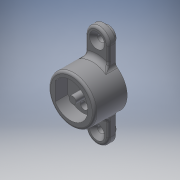
# Autodesk Inventor part: cycloid_input_cam_motor_adapter
Saved by Autodesk Inventor 2019.4 (Build 234330000, 330)
## iProperties
Created: 2019-09-11
Part Number: cycloid_input_cam_motor_adapter
Material: Generic
Document SubType Name: Modeling
Designer: cdi
Density: 1 g/cm^3
Appearance: Default
Author: cdi
Autodesk Inventor part; units mm, degrees
ref_plane "YZ Plane" through (0, 0, 0) normal (1, 0, 0) x (0, 1, 0)
ref_plane "XZ Plane" through (0, 0, 0) normal (0, 1, 0) x (-1, 0, 0)
ref_plane "XY Plane" through (0, 0, 0) normal (0, 0, 1) x (1, 0, 0)
sketch "Sketch1" plane through (0, 0, 0) normal (0, 0, 1) x (1, 0, 0)
  circle A0 centre (0, 0) radius 10
  dimension "d0" = 20
  constraints: 1 centre point, 1 coincident
  measures "d0" diameter of A0
extrude "Extrusion1" add sketch "Sketch1" along normal blind 8.5
sketch "Sketch2" plane through (0, 0, 8.5) normal (0, 0, 1) x (1, 0, 0)
  circle A0 centre (0, 0) radius 1.5
  dimension "d3" = 3
  constraints: 1 centre point, 1 coincident
  measures "d3" diameter of A0
extrude "Extrusion2" add sketch "Sketch2" along normal blind 5
chamfer "Chamfer1" distance 0.4 angle 45 1 edges at (-1.5, 0, 8.5)
sketch "Sketch3" plane through (0, 0, 8.5) normal (0, 0, 1) x (1, 0, 0)
  circle A0 centre (-0.5, 0) radius 7.575
  circle A1 centre (0, 0) radius 10 projected
  line L0 (0, 0) -> (-7.1422, 0)
  dimension "d9" = 15.15
  dimension "d25" = 0.5
  constraints: 2 end point, 1 centre point, 1 horizontal, 1 point on line
  measures "d9" diameter of A0
  measures "d25" distance of point (0, 0) A0.centre
extrude "Extrusion3" add sketch "Sketch3" along normal blind 5.5
sketch "Sketch4" plane through (0, 0, 0) normal (0, 0, -1) x (-1, 0, 0)
  circle A0 centre (0, 4.5) radius 1.5
  point P0 (0, 0)
  dimension "d13" = 4.5
  dimension "d14" = 3
  constraints: 1 centre point
  measures "d13" distance of point (0, 0) A0.centre
  measures "d14" diameter of A0
hole "Hole1" at (0, 4.5, 0) direction (0, 0, 1) diameter 3.25 end through all countersink diameter 6.5 countersink angle 90
pattern_circular "Circular Pattern1" count 2 over 360 about axis through (0, 0, 0) along (0, 0, 1) of "Hole1"
sketch "Sketch5" plane through (0, 0, 0) normal (0, 0, -1) x (-1, 0, 0)
  line L0 (-5, 17) -> (5, 17)
  line L1 (5, 17) -> (5, -17)
  line L2 (5, -17) -> (-5, -17)
  line L3 (-5, -17) -> (-5, 17)
  line L4 (-5, 17) -> (5, -17) construction
  line L5 (5, 17) -> (-5, -17) construction
  circle A0 centre (0, 0) radius 10 projected
  arc A1 (5, 8.6603) -> (-5, 8.6603) centre (0, 0) ccw
  arc A2 (-5, -8.6603) -> (5, -8.6603) centre (0, 0) ccw
  dimension "d26" = 10
  dimension "d27" = 34
  constraints: 12 end point, 8 point on circle, 4 point on line, 2 centre point, 2 concentric, 2 midpoint, 2 parallel, 1 horizontal, 1 perpendicular
  measures "d26" distance of L1.end L2.end
  measures "d27" distance of L0.end L1.end
extrude "Extrusion4" add sketch "Sketch5" against normal blind 3 contours L0 L1 A0 L3 | A0 L1 L2 L3
sketch "Sketch6" plane through (0, 0, 0) normal (0, 0, -1) x (-1, 0, 0)
  line L0 (-5, 17) -> (5, 17) projected
  circle A0 centre (0, 17) radius 5
  line L1 (5, -17) -> (-5, -17) projected
  circle A1 centre (0, -17) radius 5
  point P0 (0, 0)
  constraints: 2 horizontal alignment, 2 midpoint, 4 other
extrude "Extrusion5" add sketch "Sketch6" against normal blind 3
sketch "Sketch7" plane through (0, 0, 0) normal (0, 0, -1) x (-1, 0, 0)
  arc A0 (5, 17) -> (-5, 17) centre (0, 17) ccw projected
  circle A1 centre (0, 17) radius 3.25
  arc A2 (-5, -17) -> (5, -17) centre (0, -17) ccw projected
  circle A3 centre (0, -17) radius 3.25
  point P0 (0, 0)
  dimension "d32" = 6.5
  dimension "d33" = 6.5
  constraints: 2 centre point, 2 coincident
  measures "d32" diameter of A1
  measures "d33" diameter of A3
extrude "Extrusion6" add sketch "Sketch7" along normal blind 2
sketch "Sketch8" plane through (0, 0, 3) normal (0, 0, 1) x (1, 0, 0)
  arc A0 (5, 17) -> (-5, 17) centre (0, 17) ccw projected
  arc A1 (-5, -17) -> (5, -17) centre (0, -17) ccw projected
  point P0 (0, 0)
hole "Hole2" at (0, 17, 3) at (0, -17, 3) direction (0, 0, -1) diameter 3.1 end through all countersink diameter 6.5 countersink angle 90
fillet "Fillet1" radius 2 6 edges at (0, 10, 3) (5, 8.6603, 1.5) (5, -8.6603, 1.5) (0, -10, 3) (-5, -8.6603, 1.5) (-5, 8.6603, 1.5)
fillet "Fillet2" radius 1 2 edges at (3.25, 17, 0) (3.25, -17, 0)
fillet "Fillet3" radius 1 1 edges at (-10, 0, 14)
fillet "Fillet4" radius 1 14 edges at (-5, 13.9544, 3) (-5, 10.3092, 3.0749) (-5.256, 8.7679, 4.0831) (5, 13.9544, 3) (5, 10.3092, 3.0749) (5.256, 8.7679, 4.0831) (0, 22, 3) (5, -13.9544, 3) (5, -10.3092, 3.0749) (5.256, -8.7679, 4.0831) (-5, -13.9544, 3) (-5, -10.3092, 3.0749) (-5.256, -8.7679, 4.0831) (0, -22, 3)
sketch "Sketch10" plane through (-0.5, 0, 8.5) normal (0, 0, 1) x (1, 0, 0)
  circle A0 centre (0.5, -4.5) radius 1.625 projected
  circle A1 centre (0.5, 4.5) radius 1.625 projected
  circle A2 centre (0, 0) radius 7.575 projected
  circle A3 centre (0.5, 0) radius 1.9 projected
  line L0 (0.5, -4.5) -> (0.5, 4.5)
  line L1 (-6.5, -3.8898) -> (-6.5, 3.8898)
  dimension "d50" = 7
  constraints: 4 end point, 2 point on circle, 1 parallel, 1 vertical
  measures "d50" distance between parallel lines of L1 L0
extrude "Extrusion8" add sketch "Sketch10" along normal up to surface (5.5 mm away) contours L1 A2 picked at (-6.7273, -0.8028)
body "Solid1"
